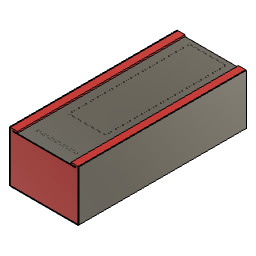
John_AlmostFinal (Autodesk Fusion 360 design; units mm, degrees)
Autodesk Fusion 360 part; units mm, degrees
sketch "Sketch1" plane through (0, 0, 0) normal (0, 1, 0) x (1, 0, 0)
  line L0 (-42.5, -60) -> (42.5, -60)
  line L1 (42.5, -60) -> (42.5, 0)
  line L2 (42.5, 0) -> (-42.5, 0)
  line L3 (-42.5, 0) -> (-42.5, -60)
  dimension "d1" = 85
  dimension "d2" = 60
  constraint horizontal L0
  constraint vertical L1
  constraint horizontal L2
  constraint vertical L3
  constraint midpoint L2 origin
  measures "d1" distance of L0.start L0.end
  measures "d2" distance of L0.start L2.end
extrude "Extrude1" add sketch "Sketch1" along normal blind 210 makes body 1
sketch "Sketch2" plane through (0, 0, 0) normal (0, 0, 1) x (1, 0, 0)
  line L0 (41, 45.5) -> (-41, 45.5)
  line L1 (-41, 45.5) -> (-41, 1.5)
  line L2 (-41, 1.5) -> (41, 1.5)
  line L3 (41, 1.5) -> (41, 45.5)
  line L4 (42.5, 0) -> (-42.5, 0)
  point P0 (0, 1.5)
  dimension "d5" = 82
  dimension "d6" = 44
  dimension "d7" = 1.5
  constraint horizontal L0
  constraint vertical L1
  constraint horizontal L2
  constraint vertical L3
  constraint midpoint L2 P0
  constraint vertical origin P0
  measures "d5" distance of L0.start L0.end
  measures "d6" distance of L0.start L2.end
  measures "d7" distance of L2.end L4
extrude "Extrude2" cut sketch "Sketch2" along normal blind 58 bodies 1
sketch "Sketch3" plane through (0, 0, 0) normal (0, 0, 1) x (1, 0, 0)
  line L0 (-25, 15) -> (25, 15)
  line L1 (25, 15) -> (25, 17.5)
  line L2 (25, 17.5) -> (-25, 17.5)
  line L3 (-25, 17.5) -> (-25, 15)
  point P0 (0, 17.5)
  dimension "d10" = 50
  dimension "d11" = 2.5
  constraint horizontal L0
  constraint vertical L1
  constraint horizontal L2
  constraint vertical L3
  constraint midpoint L2 P0
  constraint vertical origin P0
  measures "d10" distance of L0.start L0.end
  measures "d11" distance of L0.start L2.end
extrude "Extrude3" cut sketch "Sketch3" along normal blind 60 bodies 1
sketch "Sketch4" plane through (0, 0, 0) normal (0, 0, 1) x (1, 0, 0)
  line L0 (23.5, 53.4144) -> (-23.5, 53.4144)
  line L1 (-23.5, 53.4144) -> (-23.5, 205.4144)
  line L2 (-23.5, 205.4144) -> (23.5, 205.4144)
  line L3 (23.5, 205.4144) -> (23.5, 53.4144)
  point P0 (0, 53.4144)
  point P1 (-23.5, 129.4144)
  dimension "d14" = 47
  dimension "d15" = 152
  constraint horizontal L0
  constraint vertical L1
  constraint horizontal L2
  constraint vertical L3
  constraint midpoint L0 P0
  constraint vertical origin P0
  constraint midpoint L1 P1
  measures "d14" distance of L0.start L0.end
  measures "d15" distance of L0.start L2.end
extrude "Extrude4" cut sketch "Sketch4" against normal blind 25 from surface at 60 bodies 1
sketch "Sketch5" plane through (0, 0, 0) normal (0, -1, 0) x (1, 0, 0)
  line L0 (-42.5, 60) -> (-42.5, 0)
  line L1 (-42.5, 0) -> (42.5, 0)
  line L2 (42.5, 0) -> (42.5, 60)
  line L3 (42.5, 60) -> (-42.5, 60)
  line L4 (-39.5, 60) -> (39.5, 60)
  line L5 (-39.5, 60) -> (-39.5, 61)
  line L6 (-39.5, 61) -> (-33.5, 61)
  line L7 (-33.5, 61) -> (-33.5, 63)
  line L8 (-33.5, 63) -> (-42.5, 63)
  line L9 (-42.5, 60) -> (-39.5, 60)
  line L10 (-42.5, 63) -> (-42.5, 60)
  line L11 (39.5, 60) -> (39.5, 61)
  line L12 (39.5, 61) -> (33.5, 61)
  line L13 (33.5, 61) -> (33.5, 63)
  line L14 (33.5, 63) -> (42.5, 63)
  line L15 (42.5, 60) -> (42.5, 63)
  point P0 (42.5, 60)
  dimension "d19" = 1
  dimension "d20" = 6
  dimension "d21" = 2
  dimension "d22" = 9
  dimension "d23" = 3
  dimension "d24" = 1
  dimension "d25" = 6
  dimension "d26" = 2
  dimension "d27" = 9
  dimension "d28" = 3
  constraint coincident L3 L4.start
  constraint coincident L3 L4.end
  constraint perpendicular L4 L5
  constraint perpendicular L5 L6
  constraint perpendicular L6 L7
  constraint perpendicular L7 L8
  constraint coincident L0.start L3.end
  constraint perpendicular L5 L9
  constraint perpendicular L4 L11
  constraint perpendicular L11 L12
  constraint perpendicular L12 L13
  constraint perpendicular L13 L14
  constraint coincident P0 L2.end
  measures "d19" distance of L4.start L5.end
  measures "d20" distance of L5.end L6.end
  measures "d21" distance of L6.end L7.end
  measures "d22" distance of L7.end L8.end
  measures "d23" distance of L0.start L4.start
  measures "d24" distance of L4.end L11.end
  measures "d25" distance of L11.end L12.end
  measures "d26" distance of L12.end L13.end
  measures "d27" distance of L13.end L14.end
  measures "d28" distance of L4.end P0
extrude "Extrude5" add sketch "Sketch5" against normal blind 210 contours L3 L5 L6 L7 L8 L9 L10 | L3 L11 L12 L13 L14 L15 bodies 1
sketch "Sketch7" plane through (0, 0, 0) normal (0, 1, 0) x (1, 0, 0)
  line L0 (-39.5093, -59.9435) -> (39.4907, -59.9435)
  line L1 (39.4907, -59.9435) -> (39.4907, -60.9435)
  line L2 (39.4907, -60.9435) -> (-39.5093, -60.9435)
  line L3 (-39.5093, -60.9435) -> (-39.5093, -59.9435)
  dimension "d31" = 79
  dimension "d32" = 1
  constraint horizontal L0
  constraint vertical L1
  constraint horizontal L2
  constraint vertical L3
  measures "d31" distance of L0.start L0.end
  measures "d32" distance of L0.start L2.end
extrude "Extrude6" add sketch "Sketch7" along normal blind 210 separate body makes body 2
sketch "Sketch8" plane through (0, 0, 0) normal (0, 0, 1) x (1, 0, 0)
  line L0 (22.5, 54.4144) -> (-22.5, 54.4144)
  line L1 (-22.5, 54.4144) -> (-22.5, 204.4144)
  line L2 (-22.5, 204.4144) -> (22.5, 204.4144)
  line L3 (22.5, 204.4144) -> (22.5, 54.4144)
  point P0 (0, 54.4144)
  point P1 (-22.5, 129.4144)
  point P2 (-23.5, 129.4144)
  point P3 (0, 53.4144)
  dimension "d35" = 45
  dimension "d36" = 150
  constraint horizontal L0
  constraint vertical L1
  constraint horizontal L2
  constraint vertical L3
  constraint midpoint L0 P0
  constraint midpoint L1 P1
  constraint horizontal P1 P2
  constraint vertical P0 P3
  measures "d35" distance of L0.start L0.end
  measures "d36" distance of L0.start L2.end
extrude "Extrude7" add sketch "Sketch8" along normal blind 25 from surface at 35 separate body makes body 3
sketch "Sketch9" plane through (0, 0, 0) normal (0, 1, 0) x (1, 0, 0)
  line L0 (-42.5, -63.0489) -> (42.5, -63.0489)
  line L1 (42.5, -63.0489) -> (42.5, -0.0489)
  line L2 (42.5, -0.0489) -> (-42.5, -0.0489)
  line L3 (-42.5, -0.0489) -> (-42.5, -63.0489)
  point P0 (0, -63.0489)
  dimension "d54" = 85
  dimension "d55" = 63
  constraint horizontal L0
  constraint vertical L1
  constraint horizontal L2
  constraint vertical L3
  constraint midpoint L0 P0
  constraint vertical P0 origin
  measures "d54" distance of L0.start L0.end
  measures "d55" distance of L0.start L2.end
extrude "Extrude12" add sketch "Sketch9" along normal blind 210 separate body makes body 4
shell "Shell3" thickness 1 outward yes removed faces 1 at (-14.1667, 140, 63.0489) on bodies 4
extrude "Extrude13" cut 1 faces at (-14.5, -1, 20.3823) along direction (0, 1, 0) blind 1 on bodies 4 bodies 4
extrude "Extrude14" cut 1 faces at (-14.5, 211, 20.3823) along direction (0, -1, 0) blind 1 on bodies 4 bodies 4
fillet "Fillet3" radius 1 2 edges at (-43.5, 105, -0.9511) (43.5, 105, -0.9511) on bodies 4
equation "d37 = 60 mm - 25 mm"
